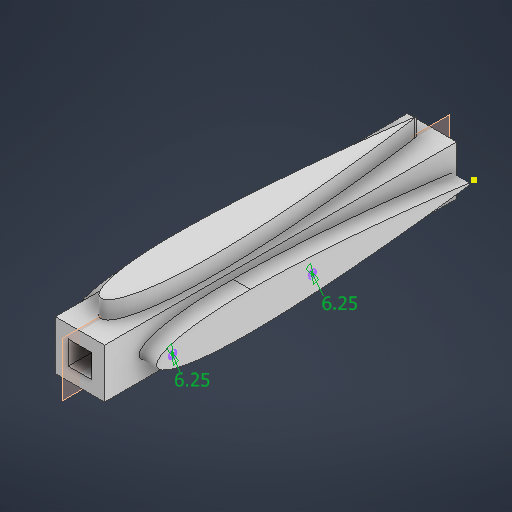
# Autodesk Inventor part: Part2
Saved by Autodesk Inventor 2025.1 (Build 291241000, 241)
## iProperties
Created: 2025-01-31
Part Number: Part2
Material: Generic
Document SubType Name: Modeling
Designer: Shane
Density: 1 g/cm^3
Appearance: Default
Author: Shane
Autodesk Inventor part; units mm, degrees
ref_plane "YZ Plane" through (0, 0, 0) normal (1, 0, 0) x (0, 1, 0)
ref_plane "XZ Plane" through (0, 0, 0) normal (0, 1, 0) x (-1, 0, 0)
ref_plane "XY Plane" through (0, 0, 0) normal (0, 0, 1) x (1, 0, 0)
sketch "Sketch1" plane through (0, 0, 0) normal (0, 0, 1) x (1, 0, 0)
  line L0 (-21, 21) -> (21, 21)
  line L1 (21, 21) -> (21, -21)
  line L2 (21, -21) -> (-21, -21)
  line L3 (-21, -21) -> (-21, 21)
  line L4 (-21, 21) -> (21, -21) construction
  line L5 (21, 21) -> (-21, -21) construction
  point P0 (0, 0)
  dimension "d0" = 42
  dimension "d1" = 42
  constraints: 12 end point, 2 midpoint, 2 parallel, 1 horizontal, 1 perpendicular
  measures "d0" distance of L0.start L0.end
  measures "d1" distance of L0.end L1.end
extrude "Extrusion1" add sketch "Sketch1" along normal blind 300
sketch "Sketch2" plane through (0, 0, 300) normal (0, 0, 1) x (1, 0, 0)
  line L0 (-21, -21) -> (21, -21) construction
  line L1 (21, -21) -> (21, 21) construction
  line L2 (21, 21) -> (-21, 21) construction
  line L3 (-21, 21) -> (-21, -21) construction
  line L4 (-10, 10) -> (10, 10)
  line L5 (10, 10) -> (10, -10)
  line L6 (10, -10) -> (-10, -10)
  line L7 (-10, -10) -> (-10, 10)
  point P0 (0, 0)
  constraints: 8 end point, 3 other
extrude "Extrusion2" cut sketch "Sketch2" against normal blind 100
sketch "Sketch3" plane through (21, -21, 0) normal (1, 0, 0) x (0, 0, -1)
  line L0 (-190.6047, 35.8888) -> (-196.449, 35.8888) construction
  line L1 (-196.449, 35.8888) -> (-202.1559, 35.8888) construction
  line L2 (-202.1559, 35.8888) -> (-207.7108, 35.7375) construction
  line L3 (-207.7108, 35.7375) -> (-213.1014, 35.5232) construction
  line L4 (-213.1014, 35.5232) -> (-218.3151, 35.2456) construction
  line L5 (-218.3151, 35.2456) -> (-223.3397, 34.9047) construction
  line L6 (-223.3397, 34.9047) -> (-228.1635, 34.5009) construction
  line L7 (-228.1635, 34.5009) -> (-232.7751, 34.0351) construction
  line L8 (-232.7751, 34.0351) -> (-237.1639, 33.5087) construction
  line L9 (-237.1639, 33.5087) -> (-241.3196, 32.9234) construction
  line L10 (-241.3196, 32.9234) -> (-245.2324, 32.2812) construction
  line L11 (-245.2324, 32.2812) -> (-248.8933, 31.5847) construction
  line L12 (-248.8933, 31.5847) -> (-252.2936, 30.8363) construction
  line L13 (-252.2936, 30.8363) -> (-255.4256, 30.039) construction
  line L14 (-255.4256, 30.039) -> (-258.2817, 29.1956) construction
  line L15 (-258.2817, 29.1956) -> (-260.8554, 28.3093) construction
  line L16 (-260.8554, 28.3093) -> (-263.1406, 27.383) construction
  line L17 (-263.1406, 27.383) -> (-265.1321, 26.4196) construction
  line L18 (-265.1321, 26.4196) -> (-266.8251, 25.422) construction
  line L19 (-266.8251, 25.422) -> (-268.2157, 24.3927) construction
  line L20 (-268.2157, 24.3927) -> (-269.3007, 23.334) construction
  line L21 (-269.3007, 23.334) -> (-270.0775, 22.248) construction
  line L22 (-270.0775, 22.248) -> (-270.5443, 21.1362) construction
  line L23 (-270.5443, 21.1362) -> (-270.7, 20) construction
  line L24 (-270.7, 20) -> (-270.5443, 18.8638) construction
  line L25 (-270.5443, 18.8638) -> (-270.0775, 17.752) construction
  line L26 (-270.0775, 17.752) -> (-269.3007, 16.666) construction
  line L27 (-269.3007, 16.666) -> (-268.2157, 15.6073) construction
  line L28 (-268.2157, 15.6073) -> (-266.8251, 14.578) construction
  line L29 (-266.8251, 14.578) -> (-265.1321, 13.5804) construction
  line L30 (-265.1321, 13.5804) -> (-263.1406, 12.617) construction
  line L31 (-263.1406, 12.617) -> (-260.8554, 11.6907) construction
  line L32 (-260.8554, 11.6907) -> (-258.2817, 10.8044) construction
  line L33 (-258.2817, 10.8044) -> (-255.4256, 9.961) construction
  line L34 (-255.4256, 9.961) -> (-252.2936, 9.1637) construction
  line L35 (-252.2936, 9.1637) -> (-248.8933, 8.4153) construction
  line L36 (-248.8933, 8.4153) -> (-245.2324, 7.7188) construction
  line L37 (-245.2324, 7.7188) -> (-241.3196, 7.0766) construction
  line L38 (-241.3196, 7.0766) -> (-237.1639, 6.4913) construction
  line L39 (-237.1639, 6.4913) -> (-232.7751, 5.9649) construction
  line L40 (-232.7751, 5.9649) -> (-228.1635, 5.4991) construction
  line L41 (-228.1635, 5.4991) -> (-223.3397, 5.0953) construction
  line L42 (-223.3397, 5.0953) -> (-218.3151, 4.7544) construction
  line L43 (-218.3151, 4.7544) -> (-213.1014, 4.4768) construction
  line L44 (-213.1014, 4.4768) -> (-207.7108, 4.2625) construction
  line L45 (-207.7108, 4.2625) -> (-202.1559, 4.1112) construction
  line L46 (-202.1559, 4.1112) -> (-196.4496, 4.022) construction
  line L47 (-196.4496, 4.022) -> (-190.6053, 3.9934) construction
  line L48 (-190.6053, 3.9934) -> (-184.6365, 4.0239) construction
  line L49 (-184.6365, 4.0239) -> (-178.5574, 4.1114) construction
  line L50 (-178.5574, 4.1114) -> (-172.382, 4.2535) construction
  line L51 (-172.382, 4.2535) -> (-166.1248, 4.4475) construction
  line L52 (-166.1248, 4.4475) -> (-159.8004, 4.6905) construction
  line L53 (-159.8004, 4.6905) -> (-153.4236, 4.9795) construction
  line L54 (-153.4236, 4.9795) -> (-147.0092, 5.311) construction
  line L55 (-147.0092, 5.311) -> (-140.5722, 5.6818) construction
  line L56 (-140.5722, 5.6818) -> (-134.1278, 6.0884) construction
  line L57 (-134.1278, 6.0884) -> (-127.6908, 6.5274) construction
  line L58 (-127.6908, 6.5274) -> (-121.2764, 6.9952) construction
  line L59 (-121.2764, 6.9952) -> (-114.8996, 7.4885) construction
  line L60 (-114.8996, 7.4885) -> (-108.5752, 8.0038) construction
  line L61 (-108.5752, 8.0038) -> (-102.318, 8.5378) construction
  line L62 (-102.318, 8.5378) -> (-96.1426, 9.0873) construction
  line L63 (-96.1426, 9.0873) -> (-90.0634, 9.6491) construction
  line L64 (-90.0634, 9.6491) -> (-84.0947, 10.2201) construction
  line L65 (-84.0947, 10.2201) -> (-78.2504, 10.7973) construction
  line L66 (-78.2504, 10.7973) -> (-72.5441, 11.3777) construction
  line L67 (-72.5441, 11.3777) -> (-66.9892, 11.9586) construction
  line L68 (-66.9892, 11.9586) -> (-61.5986, 12.537) construction
  line L69 (-61.5986, 12.537) -> (-56.3849, 13.1102) construction
  line L70 (-56.3849, 13.1102) -> (-51.3603, 13.6754) construction
  line L71 (-51.3603, 13.6754) -> (-46.5365, 14.23) construction
  line L72 (-46.5365, 14.23) -> (-41.9249, 14.7713) construction
  line L73 (-41.9249, 14.7713) -> (-37.5361, 15.2967) construction
  line L74 (-37.5361, 15.2967) -> (-33.3804, 15.8034) construction
  line L75 (-33.3804, 15.8034) -> (-29.4676, 16.2891) construction
  line L76 (-29.4676, 16.2891) -> (-25.8067, 16.751) construction
  line L77 (-25.8067, 16.751) -> (-22.4063, 17.1867) construction
  line L78 (-22.4063, 17.1867) -> (-19.2744, 17.5939) construction
  line L79 (-19.2744, 17.5939) -> (-16.4183, 17.9702) construction
  line L80 (-16.4183, 17.9702) -> (-13.8446, 18.3134) construction
  line L81 (-13.8446, 18.3134) -> (-11.5594, 18.6216) construction
  line L82 (-11.5594, 18.6216) -> (-9.5679, 18.8927) construction
  line L83 (-9.5679, 18.8927) -> (-7.8749, 19.1251) construction
  line L84 (-7.8749, 19.1251) -> (-6.4843, 19.3174) construction
  line L85 (-6.4843, 19.3174) -> (-5.3993, 19.4683) construction
  line L86 (-5.3993, 19.4683) -> (-4.6225, 19.5767) construction
  line L87 (-4.6225, 19.5767) -> (-4.1557, 19.6421) construction
  line L88 (-4.1557, 19.6421) -> (-4, 19.664) construction
  line L89 (-4, 19.664) -> (-4, 20.336) construction
  line L90 (-300, 11) -> (-200, 11) projected
  line L91 (-4, 20.336) -> (-4.0776, 21.1933) construction
  line L92 (-4.0776, 21.1933) -> (-4.5448, 21.2563) construction
  line L93 (-4.5448, 21.2563) -> (-5.3221, 21.3608) construction
  line L94 (-5.3221, 21.3608) -> (-6.4078, 21.5062) construction
  line L95 (-6.4078, 21.5062) -> (-7.7994, 21.6913) construction
  line L96 (-7.7994, 21.6913) -> (-9.4936, 21.9151) construction
  line L97 (-9.4936, 21.9151) -> (-11.4864, 22.176) construction
  line L98 (-11.4864, 22.176) -> (-13.7732, 22.4725) construction
  line L99 (-13.7732, 22.4725) -> (-16.3486, 22.8026) construction
  line L100 (-16.3486, 22.8026) -> (-19.2066, 23.1642) construction
  line L101 (-19.2066, 23.1642) -> (-22.3405, 23.5554) construction
  line L102 (-22.3405, 23.5554) -> (-25.7431, 23.9738) construction
  line L103 (-25.7431, 23.9738) -> (-29.4063, 24.417) construction
  line L104 (-29.4063, 24.417) -> (-33.3216, 24.8826) construction
  line L105 (-33.3216, 24.8826) -> (-37.4798, 25.3681) construction
  line L106 (-37.4798, 25.3681) -> (-41.8712, 25.871) construction
  line L107 (-41.8712, 25.871) -> (-46.4855, 26.3887) construction
  line L108 (-46.4855, 26.3887) -> (-51.3121, 26.9187) construction
  line L109 (-51.3121, 26.9187) -> (-56.3395, 27.4582) construction
  line L110 (-56.3395, 27.4582) -> (-61.556, 28.0048) construction
  line L111 (-61.556, 28.0048) -> (-66.9495, 28.5556) construction
  line L112 (-66.9495, 28.5556) -> (-72.5074, 29.108) construction
  line L113 (-72.5074, 29.108) -> (-78.2165, 29.6593) construction
  line L114 (-78.2165, 29.6593) -> (-84.0637, 30.2066) construction
  line L115 (-84.0637, 30.2066) -> (-90.0353, 30.7471) construction
  line L116 (-90.0353, 30.7471) -> (-96.1172, 31.2778) construction
  line L117 (-96.1172, 31.2778) -> (-102.2953, 31.7957) construction
  line L118 (-102.2953, 31.7957) -> (-108.5552, 32.2978) construction
  line L119 (-108.5552, 32.2978) -> (-114.8821, 32.7808) construction
  line L120 (-114.8821, 32.7808) -> (-121.2615, 33.2414) construction
  line L121 (-121.2615, 33.2414) -> (-127.6781, 33.6765) construction
  line L122 (-127.6781, 33.6765) -> (-134.1172, 34.0825) construction
  line L123 (-134.1172, 34.0825) -> (-140.5637, 34.4562) construction
  line L124 (-140.5637, 34.4562) -> (-147.0025, 34.7941) construction
  line L125 (-147.0025, 34.7941) -> (-153.4184, 35.0928) construction
  line L126 (-153.4184, 35.0928) -> (-159.7967, 35.3491) construction
  line L127 (-159.7967, 35.3491) -> (-166.1223, 35.5598) construction
  line L128 (-166.1223, 35.5598) -> (-172.3804, 35.7218) construction
  line L129 (-172.3804, 35.7218) -> (-178.5564, 35.8324) construction
  line L130 (-178.5564, 35.8324) -> (-184.6359, 35.8888) construction
  line L131 (-184.6359, 35.8888) -> (-190.6047, 35.8888) construction
  line L132 (0, 42) -> (-300, 42) projected
  spline S0 degree 4 poles (-190.6047, 35.8888) (-196.449, 35.8888) (-202.1559, 35.8888) (-207.7108, 35.7375) (-213.1014, 35.5232) (-218.3151, 35.2456) (-223.3397, 34.9047) (-228.1635, 34.5009) (-232.7751, 34.0351) (-237.1639, 33.5087) (-241.3196, 32.9234) (-245.2324, 32.2812) (-248.8933, 31.5847) (-252.2936, 30.8363) (-255.4256, 30.039) (-258.2817, 29.1956) (-260.8554, 28.3093) (-263.1406, 27.383) (-265.1321, 26.4196) (-266.8251, 25.422) (-268.2157, 24.3927) (-269.3007, 23.334) (-270.0775, 22.248) (-270.5443, 21.1362) (-270.7, 20) (-270.5443, 18.8638) (-270.0775, 17.752) (-269.3007, 16.666) (-268.2157, 15.6073) (-266.8251, 14.578) (-265.1321, 13.5804) (-263.1406, 12.617) (-260.8554, 11.6907) (-258.2817, 10.8044) (-255.4256, 9.961) (-252.2936, 9.1637) (-248.8933, 8.4153) (-245.2324, 7.7188) (-241.3196, 7.0766) (-237.1639, 6.4913) (-232.7751, 5.9649) (-228.1635, 5.4991) (-223.3397, 5.0953) (-218.3151, 4.7544) (-213.1014, 4.4768) (-207.7108, 4.2625) (-202.1559, 4.1112) (-196.4496, 4.022) (-190.6053, 3.9934) (-184.6365, 4.0239) (-178.5574, 4.1114) (-172.382, 4.2535) (-166.1248, 4.4475) (-159.8004, 4.6905) (-153.4236, 4.9795) (-147.0092, 5.311) (-140.5722, 5.6818) (-134.1278, 6.0884) (-127.6908, 6.5274) (-121.2764, 6.9952) (-114.8996, 7.4885) (-108.5752, 8.0038) (-102.318, 8.5378) (-96.1426, 9.0873) (-90.0634, 9.6491) (-84.0947, 10.2201) (-78.2504, 10.7973) (-72.5441, 11.3777) (-66.9892, 11.9586) (-61.5986, 12.537) (-56.3849, 13.1102) (-51.3603, 13.6754) (-46.5365, 14.23) (-41.9249, 14.7713) (-37.5361, 15.2967) (-33.3804, 15.8034) (-29.4676, 16.2891) (-25.8067, 16.751) (-22.4063, 17.1867) (-19.2744, 17.5939) (-16.4183, 17.9702) (-13.8446, 18.3134) (-11.5594, 18.6216) (-9.5679, 18.8927) (-7.8749, 19.1251) (-6.4843, 19.3174) (-5.3993, 19.4683) (-4.6225, 19.5767) (-4.1557, 19.6421) (-4, 19.664) (-4, 20.336) (-4.0776, 21.1933) (-4.5448, 21.2563) (-5.3221, 21.3608) (-6.4078, 21.5062) (-7.7994, 21.6913) (-9.4936, 21.9151) (-11.4864, 22.176) (-13.7732, 22.4725) (-16.3486, 22.8026) (-19.2066, 23.1642) (-22.3405, 23.5554) (-25.7431, 23.9738) (-29.4063, 24.417) (-33.3216, 24.8826) (-37.4798, 25.3681) (-41.8712, 25.871) (-46.4855, 26.3887) (-51.3121, 26.9187) (-56.3395, 27.4582) (-61.556, 28.0048) (-66.9495, 28.5556) (-72.5074, 29.108) (-78.2165, 29.6593) (-84.0637, 30.2066) (-90.0353, 30.7471) (-96.1172, 31.2778) (-102.2953, 31.7957) (-108.5552, 32.2978) (-114.8821, 32.7808) (-121.2615, 33.2414) (-127.6781, 33.6765) (-134.1172, 34.0825) (-140.5637, 34.4562) (-147.0025, 34.7941) (-153.4184, 35.0928) (-159.7967, 35.3491) (-166.1223, 35.5598) (-172.3804, 35.7218) (-178.5564, 35.8324) (-184.6359, 35.8888) (-190.6047, 35.8888) knots 1 1 1 1 1 2 3 4 5 6 7 8 9 10 11 12 13 14 15 16 17 18 19 20 21 22 23 24 25 26 27 28 29 30 31 32 33 34 35 36 37 38 39 40 41 42 43 44 45 46 47 48 49 50 51 52 53 54 55 56 57 58 59 60 61 62 63 64 65 66 67 68 69 70 71 72 73 74 75 76 77 78 79 80 81 82 83 84 85 86 87 88 89 90 91 92 93 94 95 96 97 98 99 100 101 102 103 104 105 106 107 108 109 110 111 112 113 114 115 116 117 118 119 120 121 122 123 124 125 126 127 128 129 129 129 129 129
  point P0 (0, 21)
  constraints: 130 coincident, 2 horizontal, 1 parallel, 1 perpendicular, 1 other
extrude "Extrusion3" add sketch "Sketch3" along normal blind 14.925
ref_plane "Work Plane1" through (0, -21, 0) normal (1, 0, 0) x (0, 0, -1)
mirror "Mirror1" about plane through (0, -21, 0) normal (1, 0, 0) of "Extrusion3"
sketch "Sketch4" plane through (-21, 21, 0) normal (0, 1, 0) x (1, 0, 0)
  spline S0 degree 4 poles (20.664, -15.3) (20.6506, -15.3953) (20.5854, -15.8603) (20.4763, -16.6402) (20.2935, -17.9553) (20.1026, -19.3358) (19.8704, -21.0276) (19.6, -23.0143) (19.2923, -25.2966) (18.9496, -27.8664) (18.574, -30.7188) (18.1673, -33.8465) (17.7323, -37.2426) (17.271, -40.8988) (16.7861, -44.8067) (16.28, -48.9571) (15.7554, -53.3405) (15.2149, -57.9464) (14.6611, -62.7642) (14.0965, -67.7826) (13.5242, -72.9898) (12.9465, -78.3738) (12.3664, -83.9219) (11.7867, -89.6212) (11.2101, -95.4584) (10.6398, -101.4197) (10.0785, -107.4914) (9.5295, -113.6592) (8.9959, -119.9088) (8.481, -126.2254) (7.988, -132.5945) (7.5203, -139.001) (7.0814, -145.4301) (6.6748, -151.8668) (6.3038, -158.2959) (5.972, -164.7025) (5.6827, -171.0717) (5.4391, -177.3886) (5.2444, -183.6384) (5.1014, -189.8065) (5.0129, -195.8786) (4.9812, -201.8404) (5.0083, -207.6781) (5.096, -213.3779) (5.2455, -218.9267) (5.4578, -224.3115) (5.7331, -229.5197) (6.0715, -234.5392) (6.4725, -239.3582) (6.9352, -243.9655) (7.4581, -248.3505) (8.0395, -252.5029) (8.6773, -256.4131) (9.3689, -260.0722) (10.1118, -263.4717) (10.9028, -266.6039) (11.7391, -269.462) (12.6176, -272.0398) (13.5353, -274.3322) (14.4897, -276.335) (15.479, -278.0454) (16.5033, -279.4616) (17.5645, -280.5816) (18.6684, -281.3995) (19.8145, -281.9015) (21, -282.0688) (22.1855, -281.9015) (23.3316, -281.3995) (24.4355, -280.5816) (25.4967, -279.4616) (26.521, -278.0454) (27.5103, -276.335) (28.4647, -274.3322) (29.3824, -272.0398) (30.2609, -269.462) (31.0972, -266.6039) (31.8882, -263.4717) (32.6311, -260.0722) (33.3227, -256.4131) (33.9605, -252.5029) (34.5419, -248.3505) (35.0648, -243.9655) (35.5275, -239.3582) (35.9285, -234.5392) (36.2669, -229.5197) (36.5422, -224.3115) (36.7545, -218.9267) (36.904, -213.3779) (36.9917, -207.6781) (37.0188, -201.8404) (36.9871, -195.8786) (36.8986, -189.8065) (36.7556, -183.6384) (36.5609, -177.3886) (36.3173, -171.0717) (36.028, -164.7025) (35.6962, -158.2959) (35.3252, -151.8668) (34.9186, -145.4301) (34.4797, -139.001) (34.012, -132.5945) (33.519, -126.2254) (33.0041, -119.9088) (32.4705, -113.6592) (31.9215, -107.4914) (31.3602, -101.4197) (30.7899, -95.4584) (30.2133, -89.6212) (29.6336, -83.9219) (29.0535, -78.3738) (28.4758, -72.9898) (27.9035, -67.7826) (27.3389, -62.7642) (26.7851, -57.9464) (26.2446, -53.3405) (25.72, -48.9571) (25.2139, -44.8067) (24.729, -40.8988) (24.2677, -37.2426) (23.8327, -33.8465) (23.4261, -30.719) (23.0503, -27.866) (22.7078, -25.2975) (22.3997, -23.0124) (22.1302, -21.0318) (21.896, -19.327) (21.7092, -17.9724) (21.5512, -16.8412) (21.448, -16.0934) (21.3625, -15.4943) (21.3484, -15.3846) (21.336, -15.3) knots 0 0 0 0 0 0.0063 0.010007 0.01432 0.019151 0.024441 0.030148 0.036235 0.042672 0.049434 0.056497 0.063841 0.071448 0.079299 0.087378 0.09567 0.104159 0.112831 0.121672 0.130668 0.139808 0.149077 0.158464 0.167955 0.177539 0.187203 0.196936 0.206726 0.21656 0.226428 0.236317 0.246217 0.256114 0.265999 0.275858 0.285682 0.295458 0.305174 0.31482 0.324383 0.333852 0.343216 0.352462 0.361579 0.370555 0.379378 0.388035 0.396515 0.404804 0.412889 0.420757 0.428395 0.435788 0.442923 0.449784 0.456356 0.462627 0.468581 0.47421 0.479508 0.484483 0.489161 0.493602 0.497886 0.502114 0.506398 0.510839 0.515517 0.520492 0.52579 0.531419 0.537373 0.543644 0.550216 0.557077 0.564212 0.571605 0.579243 0.587111 0.595196 0.603485 0.611965 0.620622 0.629445 0.638421 0.647538 0.656784 0.666148 0.675617 0.68518 0.694826 0.704542 0.714318 0.724142 0.734001 0.743886 0.753783 0.763683 0.773572 0.78344 0.793274 0.803064 0.812797 0.822461 0.832045 0.841536 0.850923 0.860192 0.869332 0.878328 0.887169 0.895841 0.90433 0.912622 0.920701 0.928552 0.936159 0.943503 0.950566 0.957328 0.963765 0.969852 0.975559 0.980849 0.98568 0.989993 0.9937 0.996639 1 1 1 1 1
  line L0 (21.336, -15.3) -> (21, -13)
  line L1 (21, -13) -> (20.664, -15.3)
  point P0 (21, 0)
  point P1 (20.6421, -15.4557)
  point P2 (20.5767, -15.9225)
  point P3 (20.4683, -16.6993)
  point P4 (20.3174, -17.7843)
  point P5 (20.1251, -19.1749)
  point P6 (19.8927, -20.8679)
  point P7 (19.6216, -22.8594)
  point P8 (19.3134, -25.1446)
  point P9 (18.9702, -27.7183)
  point P10 (18.5939, -30.5744)
  point P11 (18.1867, -33.7063)
  point P12 (17.751, -37.1067)
  point P13 (17.2891, -40.7676)
  point P14 (16.8034, -44.6804)
  point P15 (16.2967, -48.8361)
  point P16 (15.7713, -53.2249)
  point P17 (15.23, -57.8365)
  point P18 (14.6754, -62.6603)
  point P19 (14.1102, -67.6849)
  point P20 (13.537, -72.8986)
  point P21 (12.9586, -78.2892)
  point P22 (12.3777, -83.8441)
  point P23 (11.7973, -89.5504)
  point P24 (11.2201, -95.3947)
  point P25 (10.6491, -101.3634)
  point P26 (10.0873, -107.4426)
  point P27 (9.5378, -113.618)
  point P28 (9.0038, -119.8752)
  point P29 (8.4885, -126.1996)
  point P30 (7.9952, -132.5764)
  point P31 (7.5274, -138.9908)
  point P32 (7.0884, -145.4278)
  point P33 (6.6818, -151.8722)
  point P34 (6.311, -158.3092)
  point P35 (5.9795, -164.7236)
  point P36 (5.6905, -171.1004)
  point P37 (5.4475, -177.4248)
  point P38 (5.2535, -183.682)
  point P39 (5.1114, -189.8574)
  point P40 (5.0239, -195.9365)
  point P41 (4.9934, -201.9053)
  point P42 (5.022, -207.7496)
  point P43 (5.1112, -213.4559)
  point P44 (5.2625, -219.0108)
  point P45 (5.4768, -224.4014)
  point P46 (5.7544, -229.6151)
  point P47 (6.0953, -234.6397)
  point P48 (6.4991, -239.4635)
  point P49 (6.9649, -244.0751)
  point P50 (7.4913, -248.4639)
  point P51 (8.0766, -252.6196)
  point P52 (8.7188, -256.5324)
  point P53 (9.4153, -260.1933)
  point P54 (10.1637, -263.5936)
  point P55 (10.961, -266.7256)
  point P56 (11.8044, -269.5817)
  point P57 (12.6907, -272.1554)
  point P58 (13.617, -274.4406)
  point P59 (14.5804, -276.4321)
  point P60 (15.578, -278.1251)
  point P61 (16.6073, -279.5157)
  point P62 (17.666, -280.6007)
  point P63 (18.752, -281.3775)
  point P64 (19.8638, -281.8443)
  point P65 (21, -282)
  point P66 (22.1362, -281.8443)
  point P67 (23.248, -281.3775)
  point P68 (24.334, -280.6007)
  point P69 (25.3927, -279.5157)
  point P70 (26.422, -278.1251)
  point P71 (27.4196, -276.4321)
  point P72 (28.383, -274.4406)
  point P73 (29.3093, -272.1554)
  point P74 (30.1956, -269.5817)
  point P75 (31.039, -266.7256)
  point P76 (31.8363, -263.5936)
  point P77 (32.5847, -260.1933)
  point P78 (33.2812, -256.5324)
  point P79 (33.9234, -252.6196)
  point P80 (34.5087, -248.4639)
  point P81 (35.0351, -244.0751)
  point P82 (35.5009, -239.4635)
  point P83 (35.9047, -234.6397)
  point P84 (36.2456, -229.6151)
  point P85 (36.5232, -224.4014)
  point P86 (36.7375, -219.0108)
  point P87 (36.8888, -213.4559)
  point P88 (36.9781, -207.7496)
  point P89 (37.0066, -201.9053)
  point P90 (36.9761, -195.9365)
  point P91 (36.8886, -189.8574)
  point P92 (36.7465, -183.682)
  point P93 (36.5525, -177.4248)
  point P94 (36.3095, -171.1004)
  point P95 (36.0205, -164.7236)
  point P96 (35.689, -158.3092)
  point P97 (35.3182, -151.8722)
  point P98 (34.9116, -145.4278)
  point P99 (34.4726, -138.9908)
  point P100 (34.0048, -132.5764)
  point P101 (33.5115, -126.1996)
  point P102 (32.9962, -119.8752)
  point P103 (32.4622, -113.618)
  point P104 (31.9127, -107.4426)
  point P105 (31.3509, -101.3634)
  point P106 (30.7799, -95.3947)
  point P107 (30.2027, -89.5504)
  point P108 (29.6223, -83.8441)
  point P109 (29.0414, -78.2892)
  point P110 (28.463, -72.8986)
  point P111 (27.8898, -67.6849)
  point P112 (27.3246, -62.6603)
  point P113 (26.77, -57.8365)
  point P114 (26.2287, -53.2249)
  point P115 (25.7033, -48.8361)
  point P116 (25.1966, -44.6804)
  point P117 (24.7109, -40.7676)
  point P118 (24.249, -37.1067)
  point P119 (23.8133, -33.7063)
  point P120 (23.4061, -30.5744)
  point P121 (23.0298, -27.7183)
  point P122 (22.6866, -25.1446)
  point P123 (22.3784, -22.8594)
  point P124 (22.1073, -20.8679)
  point P125 (21.8749, -19.1749)
  point P126 (21.6826, -17.7843)
  point P127 (21.5317, -16.6993)
  point P128 (21.4233, -15.9225)
  point P129 (21.3579, -15.4557)
  constraints: 4 end point, 132 other
extrude "Extrusion4" add sketch "Sketch4" along normal blind 14.925
sketch "Sketch5" plane through (35.925, -21, 0) normal (1, 0, 0) x (0, 0, -1)
  circle A0 centre (-257, 21) radius 3.125
  circle A1 centre (-138.006, 21) radius 3.125
  point P0 (0, 21)
  dimension "d10" = 6.25
  dimension "d11" = 6.25
  constraints: 2 centre point
  measures "d10" diameter of A0
  measures "d11" diameter of A1
equation "\"d1\" = d0"
body "Solid1"
